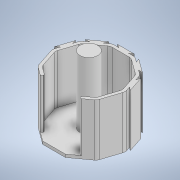
# Autodesk Inventor part: holder-10
Saved by Autodesk Inventor 2020 (Build 240168000, 168)
## iProperties
Created: 2020-02-16
Part Number: holder-10
Material: Generic
Document SubType Name: Modeling
Designer: Ball
Density: 1 g/cm^3
Appearance: Default
Author: Ball
Autodesk Inventor part; units mm, degrees
ref_plane "YZ Plane" through (0, 0, 0) normal (1, 0, 0) x (0, 1, 0)
ref_plane "XZ Plane" through (0, 0, 0) normal (0, 1, 0) x (-1, 0, 0)
ref_plane "XY Plane" through (0, 0, 0) normal (0, 0, 1) x (1, 0, 0)
sketch "Sketch1" plane through (0, 0, 0) normal (0, 1, 0) x (-1, 0, 0)
  line L0 (53.4143, 0) -> (43.2131, -31.3961)
  line L1 (43.2131, -31.3961) -> (16.5059, -50.8)
  line L2 (16.5059, -50.8) -> (-16.5059, -50.8)
  line L3 (-16.5059, -50.8) -> (-43.2131, -31.3961)
  line L4 (-43.2131, -31.3961) -> (-53.4143, 0)
  line L5 (-53.4143, 0) -> (-43.2131, 31.3961)
  line L6 (-43.2131, 31.3961) -> (-16.5059, 50.8)
  line L7 (-16.5059, 50.8) -> (16.5059, 50.8)
  line L8 (16.5059, 50.8) -> (43.2131, 31.3961)
  line L9 (43.2131, 31.3961) -> (53.4143, 0)
  point P0 (0, 0)
  point P1 (0, 0)
  dimension "d0" = 50.8
  constraints: 20 end point, 1 coincident, 21 other
  measures "d0" distance from line of L7 point (0, 0)
extrude "Extrusion1" add sketch "Sketch1" along normal blind 76.2
sketch "Sketch2" plane through (0, 76.2, 0) normal (0, 1, 0) x (1, 0, 0)
  line L0 (-48.9275, 0) -> (-39.5832, 28.7589)
  line L1 (-39.5832, 28.7589) -> (-15.1194, 46.5328)
  line L2 (-15.1194, 46.5328) -> (15.1194, 46.5328)
  line L3 (15.1194, 46.5328) -> (39.5832, 28.7589)
  line L4 (39.5832, 28.7589) -> (48.9275, 0)
  line L5 (48.9275, 0) -> (39.5832, -28.7589)
  line L6 (39.5832, -28.7589) -> (27.3513, -37.6458)
  line L7 (-27.3513, -37.6458) -> (-39.5832, -28.7589)
  line L8 (-39.5832, -28.7589) -> (-48.9275, 0)
  line L9 (-43.2131, 31.3961) -> (-53.4143, 0) projected
  line L10 (27.3513, -59.865) -> (27.3513, -37.6458)
  line L11 (-27.3513, -37.6458) -> (-27.3513, -59.865)
  line L12 (-27.3513, -59.865) -> (27.3513, -59.865)
  point P0 (0, 0)
  point P1 (0, 0)
  dimension "d3" = 4.2672
  constraints: 24 end point, 1 coincident, 1 perpendicular, 1 vertical, 16 other
  measures "d3" distance between parallel lines of L0 L9
extrude "Extrusion2" cut sketch "Sketch2" against normal blind 71.9328
fillet "Fillet1" radius 1.905 4 edges at (-27.3513, 40.2336, 42.9204) (-27.3513, 40.2336, 37.6458) (27.3513, 40.2336, 37.6458) (27.3513, 40.2336, 42.9204)
sketch "Sketch3" plane through (0, 4.2672, 0) normal (0, 1, 0) x (1, 0, 0)
  circle A0 centre (0, 0) radius 12.954
  dimension "d7" = 25.908
  constraints: 1 centre point, 1 coincident
  measures "d7" diameter of A0
extrude "Extrusion3" add sketch "Sketch3" along normal blind 97.3328
sketch "Sketch4" plane through (0, 76.2, 0) normal (0, 1, 0) x (1, 0, 0)
  line L0 (16.5059, 50.8) -> (-16.5059, 50.8) projected
  line L1 (0, 50.8) -> (7.112, 50.8)
  line L2 (0, 50.8) -> (-7.112, 50.8)
  line L3 (0, 50.8) -> (0, 54.0512)
  line L4 (0, 54.0512) -> (12.192, 54.0512)
  line L5 (0, 54.0512) -> (-12.192, 54.0512)
  line L6 (-12.192, 54.0512) -> (-7.112, 50.8)
  line L7 (7.112, 50.8) -> (12.192, 54.0512)
  line L8 (31.7705, 43.7283) -> (21.907, 50.8946)
  line L9 (21.907, 50.8946) -> (24.1058, 45.2784)
  line L10 (29.8595, 41.0981) -> (24.1058, 45.2784)
  line L11 (29.8595, 41.0981) -> (35.6132, 36.9177)
  line L12 (35.6132, 36.9177) -> (41.634, 36.5621)
  line L13 (31.7705, 43.7283) -> (41.634, 36.5621)
  line L14 (51.4057, 16.7027) -> (47.6382, 28.298)
  line L15 (47.6382, 28.298) -> (46.1159, 22.462)
  line L16 (48.3137, 15.6981) -> (46.1159, 22.462)
  line L17 (48.3137, 15.6981) -> (50.5114, 8.9341)
  line L18 (50.5114, 8.9341) -> (55.1733, 5.1075)
  line L19 (51.4057, 16.7027) -> (55.1733, 5.1075)
  line L20 (-41.634, 36.5621) -> (-35.6132, 36.9177)
  line L21 (-31.7705, 43.7283) -> (-41.634, 36.5621)
  line L22 (-29.8595, 41.0981) -> (-35.6132, 36.9177)
  line L23 (-29.8595, 41.0981) -> (-24.1058, 45.2784)
  line L24 (-31.7705, 43.7283) -> (-21.907, 50.8946)
  line L25 (-24.1058, 45.2784) -> (-21.907, 50.8946)
  line L26 (-12.192, 54.0512) -> (-7.112, 50.8)
  line L27 (0, 50.8) -> (-7.112, 50.8)
  line L28 (0, 54.0512) -> (-12.192, 54.0512)
  line L29 (0, 50.8) -> (7.112, 50.8)
  line L30 (7.112, 50.8) -> (12.192, 54.0512)
  line L31 (0, 54.0512) -> (12.192, 54.0512)
  line L32 (-48.3137, 15.6981) -> (-46.1159, 22.462)
  line L33 (-46.1159, 22.462) -> (-47.6382, 28.298)
  line L34 (-51.4057, 16.7027) -> (-47.6382, 28.298)
  line L35 (-48.3137, 15.6981) -> (-51.4057, 16.7027)
  line L36 (-48.3137, 15.6981) -> (-50.5114, 8.9341)
  line L37 (-55.1733, 5.1075) -> (-50.5114, 8.9341)
  line L38 (-51.4057, 16.7027) -> (-55.1733, 5.1075)
  point P0 (0, 0)
  dimension "d17" = 72
  dimension "d21" = 72
  constraints: 76 end point, 2 point on line, 1 horizontal, 1 midpoint, 1 parallel, 1 vertical, 63 other
extrude "Extrusion4" add sketch "Sketch4" against normal blind 76.2
fillet "Fillet2" radius 8.89 7 edges at (-48.9275, 40.2336, 0) (-15.1194, 40.2336, -46.5328) (15.1194, 40.2336, -46.5328) (-39.5832, 40.2336, -28.7589) (-39.5832, 40.2336, 28.7589) (39.5832, 40.2336, -28.7589) (48.9275, 40.2336, 0)
fillet "Fillet3" radius 8.89 8 edges at (43.2131, 38.1, 31.3961) (53.4143, 38.1, 0) (43.2131, 38.1, -31.3961) (16.5059, 38.1, -50.8) (-16.5059, 38.1, -50.8) (-43.2131, 38.1, -31.3961) (-53.4143, 38.1, 0) (-43.2131, 38.1, 31.3961)
body "Solid1"
